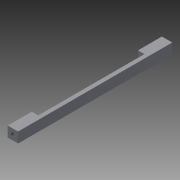
# Autodesk Inventor part: TopSupportPlate
Saved by Autodesk Inventor 2015 SP1 (Build 190203100, 203)
## iProperties
Created: 2015-08-28
Part Number: TopSupportPlate
Material: Generic
Document SubType Name: Modeling
Designer: I Rabey
Density: 1 g/cm^3
Appearance: Default
Author: I Rabey
Autodesk Inventor part; units mm, degrees
ref_plane "YZ Plane" through (0, 0, 0) normal (1, 0, 0) x (0, 1, 0)
ref_plane "XZ Plane" through (0, 0, 0) normal (0, 1, 0) x (-1, 0, 0)
ref_plane "XY Plane" through (0, 0, 0) normal (0, 0, 1) x (1, 0, 0)
sketch "Sketch1" plane through (0, 0, 0) normal (0, 1, 0) x (-1, 0, 0)
  line L0 (4, 59.5) -> (-4, 59.5)
  line L1 (-4, 59.5) -> (-4, -59.5)
  line L2 (-4, -59.5) -> (4, -59.5)
  line L3 (4, -59.5) -> (4, 59.5)
  line L4 (4, 59.5) -> (-4, -59.5) construction
  line L5 (-4, 59.5) -> (4, -59.5) construction
  point P0 (0, 0)
  dimension "d0" = 8
  dimension "d1" = 119
  constraints: 12 end point, 2 midpoint, 2 parallel, 1 horizontal, 1 perpendicular
  measures "d0" distance of L2.end L1.end
  measures "d1" distance of L1.end L0.end
extrude "Extrusion1" add sketch "Sketch1" along normal blind 8
sketch "Sketch2" plane through (0, 8, 0) normal (0, 1, 0) x (1, 0, 0)
  line L0 (-9, -41) -> (1, -41)
  line L1 (1, -41) -> (1, 41)
  line L2 (1, 41) -> (-9, 41)
  line L3 (-9, 41) -> (-9, -41)
  line L4 (-4, 59.5) -> (-4, -59.5) projected
  line L5 (-9, -41) -> (1, 41) construction
  line L6 (1, -41) -> (-9, 41) construction
  point P0 (0, 0)
  point P1 (-4, 0)
  dimension "d4" = 10
  dimension "d5" = 82
  constraints: 12 end point, 3 midpoint, 2 parallel, 1 horizontal, 1 perpendicular
  measures "d4" distance of L2.end L1.end
  measures "d5" distance of L1.end L0.end
extrude "Extrusion2" cut sketch "Sketch2" against normal blind 8
sketch "Sketch3" plane through (-4, 0, 59.5) normal (0, 0, 1) x (1, 0, 0)
  circle A0 centre (4, 4) radius 1.5
  line L0 (0, 8) -> (8, 8) projected
  line L1 (8, 0) -> (8, 8) projected
  dimension "d8" = 3
  dimension "d31" = 4
  dimension "d32" = 4
  constraints: 1 centre point
  measures "d8" diameter of A0
  measures "d31" distance from line of L0 A0.centre
  measures "d32" distance from line of L1 A0.centre
hole "Hole1" at (0, 4, 59.5) direction (0, 0, -1) diameter 3 depth 8 tip angle 118
thread "Thread1" size "M3x0.5" class "6H" standard "ANSI Metric M Profile" full length
sketch "Sketch4" plane through (4, 0, -59.5) normal (0, 0, -1) x (-1, 0, 0)
  circle A0 centre (4, 4) radius 1.5
  line L0 (0, 8) -> (8, 8) projected
  line L1 (0, 0) -> (0, 8) projected
  dimension "d19" = 3
  dimension "d33" = 4
  dimension "d34" = 4
  constraints: 1 centre point
  measures "d19" diameter of A0
  measures "d33" distance from line of L0 A0.centre
  measures "d34" distance from line of L1 A0.centre
hole "Hole2" at (0, 4, -59.5) direction (0, 0, 1) diameter 3 depth 8 tip angle 118
thread "Thread2" size "M3x0.5" class "6H" standard "ANSI Metric M Profile" full length
body "Solid1"
